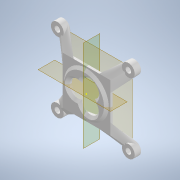
# Autodesk Inventor part: led holder
Saved by Autodesk Inventor 2021 (Build 250183000, 183)
## iProperties
Created: 2020-10-20
Part Number: led holder
Material: Generic
Document SubType Name: Modeling
Designer: VM
Density: 1 g/cm^3
Appearance: Default
Author: VM
Autodesk Inventor part; units mm, degrees
ref_plane "YZ Plane" through (0, 0, 0) normal (1, 0, 0) x (0, 1, 0)
ref_plane "XZ Plane" through (0, 0, 0) normal (0, 1, 0) x (-1, 0, 0)
ref_plane "XY Plane" through (0, 0, 0) normal (0, 0, 1) x (1, 0, 0)
sketch "Sketch1" plane through (0, 0, 0) normal (0, 0, 1) x (1, 0, 0)
  circle A0 centre (0, 0) radius 10
  circle A1 centre (4.641, 2.6795) radius 4.641
  circle A2 centre (-4.641, 2.6795) radius 4.641
  circle A3 centre (0, -5.359) radius 4.641
  circle A4 centre (0, 0) radius 12.5
  line L0 (0, -5.359) -> (0, 2.6795) construction
  point P0 (-2.3205, -1.3397)
  point P1 (2.2534, 1.4498)
  point P2 (2.3205, -1.3397)
  dimension "d0" = 20
  dimension "d1" = 25
  constraints: 3 centre point, 3 coincident, 2 end point, 1 tangent, 1 vertical, 12 other
  measures "d0" diameter of A0
  measures "d1" diameter of A4
extrude "Extrusion1" add sketch "Sketch1" along normal blind 3 contours A0 A3 A1 | A1 A2 A0 | A1 | A0 A2 A3 | A3 | A2 | A1 A3 A2 | A4
sketch "Sketch2" plane through (0, 0, 3) normal (0, 0, 1) x (1, 0, 0)
  arc A0 (2.6782, -0.083) -> (-1.2672, 2.3609) centre (2.822, 4.5558) ccw projected
  arc A1 (-1.2672, 2.3609) -> (-1.411, -2.2779) centre (-5.3564, 0.1661) ccw projected
  arc A2 (-1.411, -2.2779) -> (2.6782, -0.083) centre (2.5344, -4.7218) ccw projected
  circle A3 centre (-5.3564, 0.1661) radius 5.25
  circle A4 centre (2.822, 4.5558) radius 5.25
  circle A5 centre (2.5344, -4.7218) radius 5.25
  point P0 (0, 0)
  point P1 (-2.4279, 4.5234)
  point P2 (-2.7034, -4.3643)
  point P3 (5.1313, -0.1591)
  point P4 (-0.1065, 0.1984)
  point P5 (0.2251, -0.007)
  point P6 (-0.1186, -0.1915)
  dimension "d4" = 10.5
  dimension "d5" = 10.5
  dimension "d6" = 10.5
  constraints: 3 centre point, 3 coincident
  measures "d4" diameter of A3
  measures "d5" diameter of A4
  measures "d6" diameter of A5
extrude "Extrusion2" cut sketch "Sketch2" against normal blind 10
sketch "Sketch3" plane through (0, 0, 0) normal (0, 0, -1) x (-1, 0, 0)
  circle A0 centre (0, 0) radius 10.35
  dimension "d12" = 20.7
  constraints: 1 centre point, 1 coincident
  measures "d12" diameter of A0
extrude "Extrusion3" cut sketch "Sketch3" against normal blind 1.5
sketch "Sketch5" plane through (0, 0, 0) normal (0, 0, 1) x (1, 0, 0)
  line L0 (-15, -15) -> (15, -15)
  line L1 (15, -15) -> (15, 15)
  line L2 (15, 15) -> (-15, 15)
  line L3 (-15, 15) -> (-15, -15)
  circle A0 centre (0, 0) radius 12.5 projected
  dimension "d15" = 30
  dimension "d16" = 30
  dimension "d17" = 15
  dimension "d18" = 15
  constraints: 8 end point, 2 parallel, 1 horizontal, 1 perpendicular
  measures "d15" distance of L2.end L0.start
  measures "d16" distance of L1.end L2.end
  measures "d17" distance from line of L0 point (0, 0)
  measures "d18" distance from line of L3 point (0, 0)
extrude "Extrusion4" add sketch "Sketch5" along normal blind 1.5
chamfer "Chamfer2" distance 1.5 angle 45 3 edges at (-10.6039, 0.3287, 3) (5.0173, -9.3476, 3) (5.5866, 9.0189, 3)
chamfer "Chamfer3" distance 1.5 angle 45 1 edges at (-12.5, 0, 1.5)
ref_plane "Work Plane1" through (0, 0, -6.5) normal (0, 0, 1) x (-1, 0, 0)
sketch "Sketch6" plane through (0, 0, -6.5) normal (0, 0, 1) x (-1, 0, 0)
  circle A0 centre (22.3, 22.05) radius 1.75 projected
  circle A1 centre (22.3, -22.05) radius 1.75 projected
  circle A2 centre (-22.3, -22.05) radius 1.75 projected
  circle A3 centre (-22.3, 22.05) radius 1.75 projected
  arc A4 (-18.427, 23.05) -> (-23.3, 18.177) centre (-22.3, 22.05) ccw projected
  arc A5 (23.3, 18.177) -> (18.427, 23.05) centre (22.3, 22.05) ccw projected
  arc A6 (18.427, -23.05) -> (23.3, -18.177) centre (22.3, -22.05) ccw projected
  arc A7 (-23.3, -18.177) -> (-18.427, -23.05) centre (-22.3, -22.05) ccw projected
  circle A8 centre (22.3, 22.05) radius 4
  circle A9 centre (22.3, -22.05) radius 4
  circle A10 centre (-22.3, 22.05) radius 4
  circle A11 centre (-22.3, -22.05) radius 4
  point P0 (0, 0)
  constraints: 4 centre point, 4 coincident, 3 concentric
sketch "Sketch7" plane through (0, 0, 1.5) normal (0, 0, 1) x (1, 0, 0)
  point P0 (0, 0)
sketch "Sketch8" plane through (0, 0, 1.5) normal (0, 0, -1) x (-1, 0, 0)
  line L0 (15, -15) -> (-15, -15) projected
  line L1 (15, -15) -> (8, -15)
  line L2 (8, -15) -> (8, -8)
  line L3 (8, -8) -> (15, -8)
  line L4 (15, -8) -> (15, -15)
  point P0 (0, 0)
  dimension "d27" = 7
  dimension "d28" = 7
  constraints: 8 end point, 2 parallel, 1 horizontal, 1 perpendicular
  measures "d27" distance of L2.end L3.end
  measures "d28" distance of L1.end L2.end
loft "Loft1" add profiles "Sketch8", "Sketch6" contours all / A0 | A8 A5
sketch "Sketch9" plane through (-22.3, -22.05, -6.5) normal (0, 0, -1) x (-1, 0, 0)
  circle A0 centre (0, 0) radius 4
  point P0 (-22.3, 22.05)
  constraints: 1 centre point
extrude "Extrusion5" add sketch "Sketch9" against normal blind 4
sketch "Sketch10" plane through (-22.3, -22.05, -2.5) normal (0, 0, 1) x (1, 0, 0)
  arc A0 (1.8158, 3.5641) -> (3.6184, 1.705) centre (0, 0) ccw projected
  point P0 (22.3, 22.05)
  constraints: 1 coincident
hole "Hole1" at (-22.3, -22.05, -2.5) direction (0, 0, -1) diameter 3.5 end through all
ref_plane "Work Plane2" through (-15, 0, 0) normal (0, 1, 0) x (1, 0, 0)
mirror "Mirror1" about plane through (-15, 0, 0) normal (0, 1, 0) of "Loft1", "Extrusion5", "Hole1"
ref_plane "Work Plane3" through (0, -9.927, 0) normal (-1, 0, 0) x (0, 0, 1)
mirror "Mirror2" about plane through (0, -9.927, 0) normal (-1, 0, 0) of "Loft1", "Extrusion5", "Hole1", "Mirror1"
body "Solid1"
